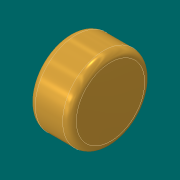
# Autodesk Inventor part: magnet
Saved by Autodesk Inventor 2016 (Build 200138000, 138)
## iProperties
Created: 2015-10-06
Part Number: magnet
Material: Brass, Soft Yellow
Document SubType Name: Modeling
Designer: Sawaiz
Density: 8.47 g/cm^3
Appearance: Brass - Satin
Author: Sawaiz
Autodesk Inventor part; units mm, degrees
ref_plane "YZ Plane" through (0, 0, 0) normal (1, 0, 0) x (0, 1, 0)
ref_plane "XZ Plane" through (0, 0, 0) normal (0, 1, 0) x (-1, 0, 0)
ref_plane "XY Plane" through (0, 0, 0) normal (0, 0, 1) x (1, 0, 0)
sketch "Sketch1" plane through (0, 0, 0) normal (1, 0, 0) x (0, 1, 0)
  circle A0 centre (0, 0) radius 3
  dimension "d0" = 6
  constraints: 1 centre point
  measures "d0" diameter of A0
extrude "Extrusion1" add sketch "Sketch1" along normal blind 3
fillet "Fillet1" radius 0.5 2 edges at (3, -3, 0) (0, -3, 0)
equation "\"d0\" = magnetDiameter"
equation "\"d1\" = magnetLength"
equation "\"materialThickness\" = 3.175"
equation "\"laserKerf\" = 0.1"
equation "\"spoolDiameter\" = 95"
equation "\"cardPinDiameter\" = 3"
equation "\"centeralShaftDiameter\" = 8"
equation "\"cardWidth\" = 85.6"
equation "\"cardHeight\" = 53.98"
equation "\"cardThickness\" = 0.76"
equation "\"cardFillet\" = 2.88"
equation "\"cardClearence\" = 0.5"
equation "\"bearingOd\" = 22"
equation "\"bearingWidth\" = 8"
equation "\"axleHeight\" = 95"
equation "\"nutTrapClearence\" = 2"
equation "\"nutTrapwidth\" = 5.5"
equation "\"nutTrapDepth\" = 2.5"
equation "\"magnetDiameter\" = 6"
equation "\"magnetLength\" = 3"
equation "\"magnetProtusion\" = 0.25"
equation "\"spoolThickness\" = 5.588"
body "Solid1"
